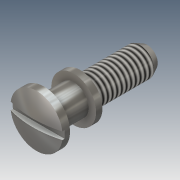
# Autodesk Inventor part: Segundo Parafuso da Ponte
Saved by Autodesk Inventor 2016 (Build 200138000, 138)
## iProperties
Created: 2018-12-01
Part Number: Segundo Parafuso da Ponte
Material: Generic
Document SubType Name: Modeling
Designer: Pedro Mendonça
Density: 1 g/cm^3
Appearance: Steel - Polished
Author: Pedro Mendonça
Autodesk Inventor part; units mm, degrees
ref_plane "YZ Plane" through (0, 0, 0) normal (1, 0, 0) x (0, 1, 0)
ref_plane "XZ Plane" through (0, 0, 0) normal (0, 1, 0) x (-1, 0, 0)
ref_plane "XY Plane" through (0, 0, 0) normal (0, 0, 1) x (1, 0, 0)
sketch "Sketch1" plane through (0, 0, 0) normal (1, 0, 0) x (0, 1, 0)
  circle A0 centre (0, 0) radius 3.85
  dimension "d0" = 7.7
  constraints: 1 centre point, 1 coincident
  measures "d0" diameter of A0
extrude "Extrusion1" add sketch "Sketch1" along normal blind 17
chamfer "Chamfer1" distance 1 distance2 2 1 edges at (0, -3.85, 0) measured on face at (0, -0.2235, 0.9948)
thread "Thread1" size "M8x1.25" class "6g" standard "ANSI Metric M Profile" full length
sketch "Sketch2" plane through (17, 0, 0) normal (1, 0, 0) x (0, 0, -1)
  circle A0 centre (0, 0) radius 3.85 projected
extrude "Extrusion2" add sketch "Sketch2" along normal blind 1 separate body
sketch "Sketch3" plane through (18, 0, 0) normal (1, 0, 0) x (0, 0, -1)
  circle A0 centre (0, 0) radius 6
  dimension "d10" = 12
  constraints: 1 centre point, 1 coincident
  measures "d10" diameter of A0
extrude "Extrusion3" add sketch "Sketch3" along normal blind 1.7 bodies 2
sketch "Sketch4" plane through (19.7, 0, 0) normal (1, 0, 0) x (0, 0, -1)
  circle A0 centre (0, 0) radius 4
  dimension "d13" = 8
  constraints: 1 centre point, 1 coincident
  measures "d13" diameter of A0
extrude "Extrusion4" add sketch "Sketch4" along normal blind 8 bodies 2
sketch "Sketch5" plane through (27.7, 0, 0) normal (1, 0, 0) x (0, 0, -1)
  circle A0 centre (0, 0) radius 7
  dimension "d16" = 14
  constraints: 1 centre point, 1 coincident
  measures "d16" diameter of A0
extrude "Extrusion5" add sketch "Sketch5" along normal blind 2 bodies 2
sketch "Sketch6" plane through (0, 0, 0) normal (0, 1, 0) x (-1, 0, 0)
  line L0 (-29.7, 7) -> (-29.7, 0)
  line L1 (-29.7, 0) -> (-30.7, 0)
  arc A0 (-29.7, 7) -> (-30.7, 0) centre (-5.7, 0) ccw
  point P0 (0, 0)
  dimension "d19" = 1
  constraints: 4 end point, 2 point on circle, 1 centre point, 1 horizontal
  measures "d19" distance of L0.end L1.end
revolve "Revolution1" add sketch "Sketch6" angle 360 about axis through (29.7, 0, 0) along (1, 0, 0) bodies 2
sketch "Sketch7" plane through (0, 0, 0) normal (0, 1, 0) x (-1, 0, 0)
  line L0 (-27.7, -7) -> (-27.7, 7) projected
  line L1 (-27.7, 0) -> (-29.1, 0) construction
  line L2 (-29.1, 0) -> (-29.1, 1) construction
  line L3 (-29.1, 1) -> (-31.1, 1)
  line L4 (-31.1, 1) -> (-31.1, -1)
  line L5 (-31.1, -1) -> (-29.1, -1)
  line L6 (-29.1, -1) -> (-29.1, 1)
  point P0 (0, 0)
  dimension "d21" = 1.4
  dimension "d22" = 1
  dimension "d23" = 2
  dimension "d24" = 2
  constraints: 12 end point, 2 horizontal, 2 parallel, 2 perpendicular, 1 midpoint
  measures "d21" distance of L1.start L1.end
  measures "d22" distance of L1.end L2.end
  measures "d23" distance of L5.end L4.end
  measures "d24" distance of L4.end L3.end
extrude "Extrusion6" cut sketch "Sketch7" along normal through all both and the other way through all bodies 2
body "Solid1"
body "Solid2"
